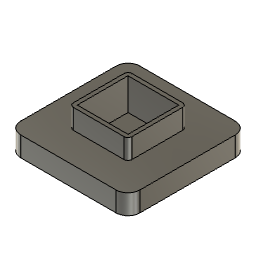
Cuvette Holder (Autodesk Fusion 360 design; units mm, degrees)
Autodesk Fusion 360 part; units mm, degrees
sketch "Sketch1" plane through (0, 0, 0) normal (0, 0, 1) x (1, 0, 0)
  line L0 (15, -15) -> (-15, -15)
  line L1 (-15, -15) -> (-15, 15)
  line L2 (-15, 15) -> (15, 15)
  line L3 (15, 15) -> (15, -15)
  line L4 (15, -15) -> (-15, 15) construction
  line L5 (-15, -15) -> (15, 15) construction
  dimension "d1" = 30
  dimension "d2" = 30
  constraint horizontal L0
  constraint perpendicular L0 L1
  constraint parallel L0 L2
  constraint parallel L1 L3
  constraint coincident L4 origin
  constraint coincident L5 origin
  measures "d1" distance of L1.end L2.end
  measures "d2" distance of L0.end L1.end
extrude "Extrude1" add sketch "Sketch1" along normal blind 5 makes body 1
sketch "Sketch2" plane through (0, 0, 5) normal (0, 0, 1) x (-1, 0, 0)
  line L0 (-15, -15) -> (15, -15)
  line L1 (15, -15) -> (15, 15)
  line L2 (15, 15) -> (-15, 15)
  line L3 (-15, 15) -> (-15, -15)
  line L4 (6.375, -6.375) -> (-6.375, -6.375)
  line L5 (-6.375, -6.375) -> (-6.375, 6.375)
  line L6 (-6.375, 6.375) -> (6.375, 6.375)
  line L7 (6.375, 6.375) -> (6.375, -6.375)
  line L8 (6.375, -6.375) -> (-6.375, 6.375) construction
  line L9 (-6.375, -6.375) -> (6.375, 6.375) construction
  line L10 (7.375, 7.375) -> (7.375, -7.375)
  line L11 (7.375, -7.375) -> (-7.375, -7.375)
  line L12 (-7.375, -7.375) -> (-7.375, 7.375)
  line L13 (-7.375, 7.375) -> (7.375, 7.375)
  dimension "d5" = 12.75
  dimension "d6" = 12.75
  dimension "d7" = -1
  constraint horizontal L4
  constraint perpendicular L4 L5
  constraint parallel L4 L6
  constraint parallel L5 L7
  constraint coincident L8 origin
  constraint coincident L9 origin
  measures "d5" distance of L5.end L6.end
  measures "d6" distance of L4.end L5.end
extrude "Extrude2" add sketch "Sketch2" along normal blind 5 contours L10 L11 L12 L13 bodies 1
extrude "Extrude3" cut 1 faces at (-2.125, -2.125, 5) along direction (0, 0, -1) up to surface (3 mm away) on bodies 1 bodies 1
fillet "Fillet1" radius 3 1 edges at (-15, 15, 2.5) on bodies 1
fillet "Fillet2" radius 3 3 edges at (-15, -15, 2.5) (15, -15, 2.5) (15, 15, 2.5) on bodies 1
fillet "Fillet3" radius 1 4 edges at (7.375, 7.375, 7.5) (-7.375, 7.375, 7.5) (7.375, -7.375, 7.5) (-7.375, -7.375, 7.5) on bodies 1
copy_body "Body->Comp1" bodies 1 removing the originals makes body 2 in component "Cuvette_Holder"
component "Cuvette_Holder" placed x (1, 0, 0) y (0, 1, 0) z (0, 0, 1) at (0, 0, 0)
